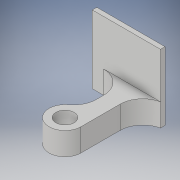
# Autodesk Inventor part: pivotholder
Saved by Autodesk Inventor 2019 (Build 230136000, 136)
## iProperties
Created: 2019-02-28
Part Number: pivotholder
Material: Generic
Document SubType Name: Modeling
Designer: erwin
Density: 1 g/cm^3
Appearance: Default
Author: erwin
Autodesk Inventor part; units mm, degrees
ref_plane "YZ Plane" through (0, 0, 0) normal (1, 0, 0) x (0, 1, 0)
ref_plane "XZ Plane" through (0, 0, 0) normal (0, 1, 0) x (-1, 0, 0)
ref_plane "XY Plane" through (0, 0, 0) normal (0, 0, 1) x (1, 0, 0)
sketch "Sketch1" plane through (0, 0, 0) normal (0, 1, 0) x (-1, 0, 0)
  circle A0 centre (0, 0) radius 4
  line L0 (0, 0) -> (0, -28) construction
  line L1 (-15, -29) -> (15, -29)
  line L2 (15, -29) -> (15, -27)
  line L3 (15, -27) -> (-15, -27)
  line L4 (-15, -27) -> (-15, -29)
  line L5 (-15, -29) -> (15, -27) construction
  line L6 (15, -29) -> (-15, -27) construction
  circle A1 centre (0, 0) radius 7
  line L7 (0, -7) -> (0, -27)
  line L8 (-7, 0) -> (-7, -27)
  dimension "d0" = 8
  dimension "d1" = 28
  dimension "d2" = 30
  dimension "d3" = 2
  dimension "d4" = 3
  constraints: 18 end point, 3 midpoint, 2 centre point, 2 parallel, 2 perpendicular, 2 point on circle, 2 point on line, 1 coincident, 1 horizontal, 1 vertical
  measures "d0" diameter of A0
  measures "d1" distance of L0.start L0.end
  measures "d2" distance of L3.end L2.end
  measures "d3" distance of L2.end L1.end
  measures "d4" radial gap between concentric circles of A0 A1
extrude "Extrusion1" add sketch "Sketch1" along normal blind 10
sketch "Sketch2" plane through (0, 10, 0) normal (0, 1, 0) x (1, 0, 0)
  line L0 (15, 29) -> (-15, 29) projected
  line L1 (7, 27) -> (15, 27) projected
  line L2 (-15, 29) -> (15, 29)
  line L3 (15, 29) -> (15, 27)
  line L4 (15, 27) -> (-15, 27)
  line L5 (-15, 27) -> (-15, 29)
  point P0 (0, 0)
  constraints: 8 end point, 2 parallel, 1 horizontal, 1 perpendicular
extrude "Extrusion2" add sketch "Sketch2" along normal blind 20
fillet "Fillet1" radius 10 3 edges at (7, 5, -27) (0, 5, -27) (0, 5, -7)
body "Solid1"
